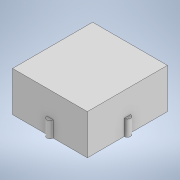
# Autodesk Inventor part: cajapic
Saved by Autodesk Inventor 2021 (Build 250183000, 183)
## iProperties
Created: 2024-01-19
Part Number: cajapic
Material: Generic
Document SubType Name: Modeling
Designer: MARCO BRAVO
Density: 1 g/cm^3
Appearance: Default
Author: MARCO BRAVO
Autodesk Inventor part; units mm, degrees
ref_plane "YZ Plane" through (0, 0, 0) normal (1, 0, 0) x (0, 1, 0)
ref_plane "XZ Plane" through (0, 0, 0) normal (0, 1, 0) x (-1, 0, 0)
ref_plane "XY Plane" through (0, 0, 0) normal (0, 0, 1) x (1, 0, 0)
sketch "Sketch1" plane through (0, 0, 0) normal (0, 1, 0) x (-1, 0, 0)
  line L0 (70, -85) -> (5, -85)
  line L1 (5, -85) -> (5, -15)
  line L2 (5, -15) -> (70, -15)
  line L3 (70, -15) -> (70, -85)
  line L4 (73, -15) -> (73, -85)
  line L5 (73, -85) -> (73, -88)
  line L6 (73, -88) -> (5, -88)
  line L7 (5, -88) -> (2, -88)
  line L8 (2, -88) -> (2, -15)
  line L9 (2, -15) -> (2, -12)
  line L10 (2, -12) -> (73, -12)
  line L11 (73, -12) -> (73, -15)
  line L12 (70, -85) -> (5, -85)
  line L13 (5, -85) -> (5, -15)
  line L14 (5, -15) -> (70, -15)
  line L15 (70, -15) -> (70, -85)
  line L16 (73, -88) -> (2, -88)
  line L17 (2, -88) -> (2, -12)
  line L18 (2, -12) -> (73, -12)
  line L19 (73, -12) -> (73, -88)
  point P0 (0, 0)
  dimension "d25" = 70
  constraints: 40 end point, 5 parallel, 5 perpendicular, 4 point on line, 2 horizontal, 1 vertical
  measures "d25" distance of L2.end L0.start
extrude "Extrusion1" add sketch "Sketch1" against normal blind 35
sketch "Sketch2" plane through (0, 0, 0) normal (0, 1, 0) x (1, 0, 0)
  line L0 (-2, 12) -> (-2, 88) projected
  line L1 (-2, 12) -> (-73, 12)
  line L2 (-73, 12) -> (-73, 88)
  line L3 (-73, 88) -> (-2, 88)
  line L4 (-2, 88) -> (-2, 12)
  point P0 (0, 0)
  constraints: 8 end point, 2 parallel, 1 horizontal, 1 perpendicular
extrude "Extrusion2" add sketch "Sketch2" along normal blind 3
sketch "Sketch3" plane through (0, -35, 0) normal (0, -1, 0) x (1, 0, 0)
  line L0 (-73, -12) -> (-2, -12) projected
  circle A0 centre (-37.5, -12) radius 3
  line L1 (-73, -88) -> (-2, -88) projected
  circle A1 centre (-37.5, -88) radius 3
  line L2 (-73, -12) -> (-73, -88) projected
  circle A2 centre (-73, -50) radius 3
  line L3 (-2, -88) -> (-2, -12) projected
  circle A3 centre (-2, -50) radius 3
  point P0 (0, 0)
  point P1 (-34.5, -88)
  point P2 (-40.5, -88)
  point P3 (-73, -53)
  point P4 (-73, -47)
  dimension "d34" = 6
  dimension "d35" = 6
  dimension "d36" = 6
  dimension "d37" = 6
  constraints: 4 centre point, 4 midpoint
  measures "d34" diameter of A0
  measures "d35" diameter of A1
  measures "d36" diameter of A2
  measures "d37" diameter of A3
extrude "Extrusion3" add sketch "Sketch3" against normal blind 15 contours A0 L0 | L0 A0 | A3 L3 | L3 A3 | L2 A2 | A1 L1 picked at (-73.9927, -50.1205) picked at (-37.3795, -88.9927)
sketch "Sketch4" plane through (0, -35, 0) normal (0, -1, 0) x (1, 0, 0)
  line L0 (-73, -88) -> (-73, -12) projected
  circle A0 centre (-73, -50) radius 1.5
  arc A1 (-34.5, -12) -> (-40.5, -12) centre (-37.5, -12) ccw projected
  circle A2 centre (-37.5, -12) radius 1.5
  circle A3 centre (-37.5, -87.9085) radius 1.5
  line L1 (-2, -12) -> (-2, -88) projected
  circle A4 centre (-2, -50) radius 1.5
  point P0 (0, 0)
  dimension "d40" = 3
  dimension "d41" = 3
  dimension "d42" = 3
  dimension "d43" = 3
  constraints: 4 centre point, 2 midpoint, 1 coincident
  measures "d40" diameter of A0
  measures "d41" diameter of A2
  measures "d42" diameter of A3
  measures "d43" diameter of A4
extrude "Extrusion4" cut sketch "Sketch4" against normal blind 7
body "Solid1"
